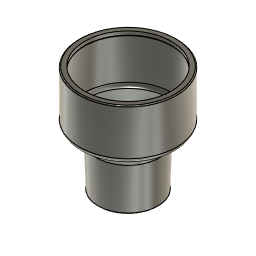
ByrnesSanderCycloneAttachment (Autodesk Fusion 360 design; units mm, degrees)
Autodesk Fusion 360 part; units mm, degrees
sketch "Sketch1" plane through (0, 0, 0) normal (0, 0, 1) x (1, 0, 0)
  circle A0 centre (0, 0) radius 15.621
  dimension "d1" = 31.242
  constraint coincident A0.centre origin
  measures "d1" diameter of A0
ref_plane "WorkPlane1" through (0, 0, 25.4) normal (0, 0, 1) x (1, 0, 0)
sketch "Sketch2" plane through (0, 0, 25.4) normal (0, 0, 1) x (1, 0, 0)
  circle A0 centre (0, 0) radius 16.383
  dimension "d3" = 32.766
  constraint coincident A0.centre origin
  measures "d3" diameter of A0
loft "Loft1" add profiles "Sketch2", "Sketch1" section 1 section 2 makes body 1
ref_plane "WorkPlane2" through (0, 0, 30.48) normal (0, 0, 1) x (1, 0, 0)
sketch "Sketch3" plane through (0, 0, 30.48) normal (0, 0, 1) x (1, 0, 0)
  circle A0 centre (0, 0) radius 25.4
  dimension "d5" = 50.8
  constraint coincident A0.centre origin
  measures "d5" diameter of A0
loft "Loft2" add profiles "Sketch3" section 1 face at (2.7305, 4.7294, 25.4) section 2 on bodies 1 bodies 1
fillet "Fillet1" radius 5.08 1 edges at (-15.2743, 5.9243, 25.4) on bodies 1
extrude "Extrude1" add 1 faces at (1.8419, 7.6928, 30.48) along direction (0, 0, 1) blind 25.4 on bodies 1 bodies 1
fillet "Fillet2" radius 2.54 1 edges at (-23.6811, 9.185, 30.48) on bodies 1
fillet "Fillet3" radius 0.508 1 edges at (-14.5639, -5.6488, 0) on bodies 1
fillet "Fillet4" radius 0.508 1 edges at (-23.6811, -9.185, 55.88) on bodies 1
copy_body "CopyPasteBodies1" bodies 1 makes body 2
move_body "Move1" bodies 2 to x (1, 0, 0) y (0, 1, 0) z (0, 0, 1) at (0, 0, -2.54)
move_body "Move2" bodies 2 to x (1, 0, 0) y (0, 1, 0) z (0, 0, 1) at (0, 0, 2.54)
scale "Scale1" factor 0.9 about (16.297, 0, 22.5339) bodies 2
move_body "Move3" bodies 2 to x (1, 0, 0) y (0, 1, 0) z (0, 0, 1) at (-1.524, 0, 0)
move_body "Move4" bodies 2 to x (1, 0, 0) y (0, 1, 0) z (0, 0, 1) at (0, 0, 1.524)
sketch "Sketch4" plane through (0, 0, 55.88) normal (0, 0, 1) x (-1, 0, 0)
  circle A0 centre (0, 0) radius 24.892
  circle A1 centre (0, 0) radius 22.606
  dimension "d17" = 45.212
  constraint concentric A0 A1
  measures "d17" diameter of A1
combine "Combine1" operation cut target body 1 tool bodies 2
extrude "Extrude2" cut sketch "Sketch4" against normal blind 24.13 contours A1 bodies 1
sketch "Sketch5" plane through (0, 0, 0) normal (0, 0, -1) x (1, 0, 0)
  circle A0 centre (0, 0) radius 15.128
  circle A1 centre (0, 0) radius 13.97
  dimension "d20" = 27.94
  constraint coincident A0.centre A1.centre
  measures "d20" diameter of A1
extrude "Extrude3" cut sketch "Sketch5" against normal blind 111.76 contours A1 bodies 1
